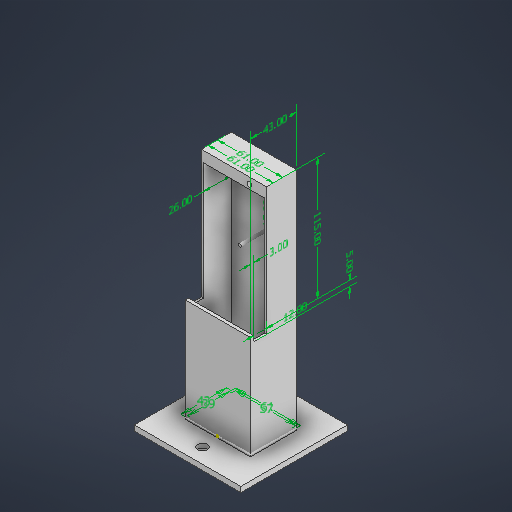
# Autodesk Inventor part: Housing of DC Motor
Saved by Autodesk Inventor 2026.2 (Build 302298010, 298A)
## iProperties
Created: 2026-04-18
Part Number: Housing of DC Motor
Material: Generic
Document SubType Name: Modeling
Designer: lenovo
Density: 1 g/cm^3
Appearance: Default
Author: lenovo
## iProperties of the stored document Housing of DC Motor_3DPrint.ipt
Created: 2026-04-19
Part Number: Housing of DC Motor_3DPrint
Material: Generic
Document SubType Name: Modeling
Designer: lenovo
Density: 1 g/cm^3
Appearance: Default
Author: lenovo
Autodesk Inventor part; units mm, degrees
ref_plane "YZ Plane" through (0, 0, 0) normal (1, 0, 0) x (0, 1, 0)
ref_plane "XZ Plane" through (0, 0, 0) normal (0, 1, 0) x (-1, 0, 0)
ref_plane "XY Plane" through (0, 0, 0) normal (0, 0, 1) x (1, 0, 0)
sketch "Sketch1" plane through (0, 0, 0) normal (0, 1, 0) x (-1, 0, 0)
  line L0 (-28.5, 19.5) -> (28.5, 19.5)
  line L1 (28.5, 19.5) -> (28.5, -19.5)
  line L2 (28.5, -19.5) -> (-28.5, -19.5)
  line L3 (-28.5, -19.5) -> (-28.5, 19.5)
  line L4 (-28.5, 19.5) -> (28.5, -19.5) construction
  line L5 (28.5, 19.5) -> (-28.5, -19.5) construction
  line L6 (-30.5, 21.5) -> (30.5, 21.5)
  line L7 (30.5, 21.5) -> (30.5, -21.5)
  line L8 (30.5, -21.5) -> (-30.5, -21.5)
  line L9 (-30.5, -21.5) -> (-30.5, 21.5)
  line L10 (-30.5, 21.5) -> (30.5, -21.5) construction
  line L11 (30.5, 21.5) -> (-30.5, -21.5) construction
  point P0 (0, 0)
  point P1 (0, -19.5)
  point P2 (0, -21.5)
  point P3 (0, 0)
  point P4 (0, 0)
  dimension "d1" = 57
  dimension "d2" = 39
  dimension "d3" = 61
  dimension "d4" = 43
  constraints: 24 end point, 5 midpoint, 4 parallel, 2 horizontal, 2 perpendicular, 1 coincident
  measures "d1" distance of L1.end L2.end
  measures "d2" distance of L0.end L1.end
  measures "d3" distance of L7.end L8.end
  measures "d4" distance of L6.end L7.end
extrude "Extrusion2" add sketch "Sketch1" against normal blind 2 contours L0 L1 L2 L3 | L6 L7 L8 L9
extrude "Extrusion3" add sketch "Sketch1" along normal blind 200
sketch "Sketch2" plane through (0, 200, 0) normal (0, 1, 0) x (1, 0, 0)
  line L0 (-30.5, -21.5) -> (-30.5, 21.5) projected
  line L1 (30.5, -21.5) -> (-30.5, -21.5)
  line L2 (-30.5, -21.5) -> (-30.5, 21.5)
  line L3 (-30.5, 21.5) -> (30.5, 21.5)
  line L4 (30.5, 21.5) -> (30.5, -21.5)
  line L5 (30.5, -21.5) -> (-30.5, 21.5) construction
  line L6 (-30.5, -21.5) -> (30.5, 21.5) construction
  point P0 (0, 0)
  constraints: 12 end point, 2 midpoint, 2 parallel, 1 horizontal, 1 perpendicular
extrude "Extrusion4" add sketch "Sketch2" along normal blind 10
sketch "Sketch6" plane through (0, -2, 0) normal (0, -1, 0) x (1, 0, 0)
  line L0 (-30.5, -21.5) -> (30.5, -21.5)
  line L1 (30.5, -21.5) -> (30.5, 21.5)
  line L2 (30.5, 21.5) -> (-30.5, 21.5)
  line L3 (-30.5, 21.5) -> (-30.5, -21.5)
  line L4 (-30.5, -21.5) -> (30.5, 21.5) construction
  line L5 (30.5, -21.5) -> (-30.5, 21.5) construction
  line L6 (-50, -50) -> (50, -50)
  line L7 (50, -50) -> (50, 50)
  line L8 (50, 50) -> (-50, 50)
  line L9 (-50, 50) -> (-50, -50)
  line L10 (-50, -50) -> (50, 50) construction
  line L11 (50, -50) -> (-50, 50) construction
  circle A0 centre (0, 0) radius 7.25
  dimension "d27" = 100
  dimension "d28" = 100
  constraints: 24 end point, 4 midpoint, 4 parallel, 2 horizontal, 2 perpendicular, 1 centre point, 1 coincident
  measures "d27" distance of L8.end L7.end
  measures "d28" distance of L7.end L6.end
extrude "Extrusion8" add sketch "Sketch6" along normal blind 5 contours L9 L8 L7 L6
extrude "Extrusion9" add sketch "Sketch6" along normal blind 5 contours L3 L2 L1 L0
extrude "Extrusion11" cut sketch "Sketch1" against normal blind 7 contours L0 L1 L2 L3
sketch "Sketch9" plane through (-30.5, 210, 21.5) normal (0, 0, 1) x (1, 0, 0)
  point P0 (30.5, -210)
sketch "Sketch10" plane through (-30.5, 210, 21.5) normal (0, 0, 1) x (1, 0, 0)
  line L0 (0, 0) -> (61, 0) projected
  line L1 (0, 0) -> (61, 0)
  line L2 (61, 0) -> (61, -120)
  line L3 (61, -120) -> (0, -120)
  line L4 (0, -120) -> (0, 0)
  line L5 (0, -120) -> (0, -115)
  line L6 (0, -115) -> (61, -115)
  point P0 (30.5, -210)
  dimension "d95" = 1.5
  dimension "d57" = 120
  dimension "d58" = 5
  constraints: 12 end point, 4 perpendicular, 2 point on line, 1 horizontal
  measures "d57" distance of L0.end L2.end
  measures "d58" distance of L3.end L5.end
extrude "Extrusion12" cut sketch "Sketch10" against normal blind 15
extrude "Extrusion13" add sketch "Sketch10" against normal blind 3 contours L6 L2 L3 L4
sketch "Sketch11" plane through (30.5, 210, -21.5) normal (0, 0, -1) x (-1, 0, 0)
  line L0 (0, 0) -> (0, -120) projected
  point P0 (30.5, -210)
  point P1 (16, -6)
  dimension "d106" = 16
  measures "d106" distance from line of L0 point (16, -6)
hole "Hole2" at (14.5, 204, -21.5) direction (0, 0, 1) diameter 4.5 end through all counterbore diameter 7 counterbore depth 4.5
sketch "Sketch12" plane through (30.5, 210, -21.5) normal (0, 0, -1) x (-1, 0, 0)
  circle A0 centre (16, -40) radius 4
  circle A1 centre (16, -6) radius 3.5 projected
  line L0 (61, -212) -> (61, 0) projected
  line L1 (0, 0) -> (0, -212) projected
  point P0 (30.5, -210)
  point P1 (13.5, -10)
  point P2 (61, -217)
  dimension "d94" = 8
  dimension "d104" = 34
  dimension "d108" = 16
  constraints: 1 centre point
  measures "d94" diameter of A0
  measures "d104" distance of A0.centre A1.centre
  measures "d108" distance from line of L1 A0.centre
extrude "Extrusion14" cut sketch "Sketch12" against normal through all contours A0
sketch "Sketch13" plane through (-28.5, -7, -19.5) normal (0, 0, 1) x (1, 0, 0)
  circle A0 centre (43, 190) radius 1.4
  line L0 (57, 207) -> (57, 0) projected
  line L1 (41.6, 190) -> (44.4, 190)
  circle A1 centre (52, 157) radius 1.4
  circle A2 centre (34, 157) radius 1.4
  point P0 (28.5, 7)
  dimension "d101" = 2.8
  dimension "d105" = 14
  dimension "d121" = 2.8
  dimension "d122" = 2.8
  constraints: 2 centre point, 2 end point, 1 horizontal, 1 midpoint, 3 other
  measures "d105" distance from line of L0 point (43, 190)
  measures "d121" diameter of A1
  measures "d122" diameter of A2
extrude "Extrusion15" cut sketch "Sketch13" against normal blind 1 contours L1 A0 picked at (43.4531, 190.1117)
sketch "Sketch14" plane through (0, -2, 0) normal (0, 1, 0) x (1, 0, 0)
  point P0 (0, 0)
  point P1 (0, 36)
  point P2 (0, -36)
hole "Hole3" at (0, -2, -36) at (0, -2, 36) direction (0, -1, 0) diameter 4.5 end through all counterbore diameter 9 counterbore depth 4
extrude "Extrusion16" cut sketch "Sketch13" against normal blind 1 contours A1 | A2
extrude "Extrusion17" add sketch "Sketch13" along normal blind 26 contours A2
sketch "Sketch15" plane through (0, -2, 0) normal (0, 1, 0) x (1, 0, 0)
  line L0 (-50, -50) -> (-50, 50) projected
  line L1 (-50, 50) -> (50, 50) projected
  arc A0 (-50, 21.777) -> (-19.4504, 50) centre (-41.4426, 43.1597) ccw
  point P0 (0, 0)
  constraints: 2 point on circle, 2 point on line, 1 centre point
extrude "Extrusion18" cut sketch "Sketch15" against normal blind 5
body "Solid1"
